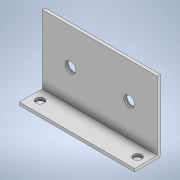
# Autodesk Inventor part: balun_support
Saved by Autodesk Inventor 2020.3 (Build 243373000, 373)
## iProperties
Created: 2021-03-09
Part Number: balun_support
Material: Generic
Document SubType Name: Modeling
Designer: Krishna Makhija
Density: 1 g/cm^3
Appearance: Default
Author: Krishna Makhija
Autodesk Inventor part; units mm, degrees
ref_plane "YZ Plane" through (0, 0, 0) normal (1, 0, 0) x (0, 1, 0)
ref_plane "XZ Plane" through (0, 0, 0) normal (0, 1, 0) x (-1, 0, 0)
ref_plane "XY Plane" through (0, 0, 0) normal (0, 0, 1) x (1, 0, 0)
sketch "Sketch1" plane through (0, 0, 0) normal (0, 0, 1) x (1, 0, 0)
  line L0 (29.994, -18.6437) -> (-29.994, -18.6437)
  line L1 (-29.994, 18.6437) -> (29.994, 18.6437)
  line L2 (29.994, -18.6437) -> (-29.994, 18.6437) construction
  line L3 (-29.994, -18.6437) -> (29.994, 18.6437) construction
  line L4 (29.994, -18.6437) -> (-29.994, -18.6437)
  line L5 (-29.994, -18.6437) -> (-29.994, -17.0588)
  line L6 (-29.994, -17.0588) -> (29.994, -17.0588)
  line L7 (29.994, -17.0588) -> (29.994, -18.6437)
  line L8 (-29.994, 18.6437) -> (-29.994, -17.0588)
  line L9 (29.994, 18.6437) -> (29.994, -17.0588)
  point P0 (0, 0)
  constraints: 20 end point, 3 parallel, 2 horizontal, 2 midpoint, 2 perpendicular, 1 vertical
extrude "Extrusion1" add sketch "Sketch1" against normal blind 1.5875 contours L6 L8 L1 L9
extrude "Extrusion2" add sketch "Sketch1" along normal blind 11.9062 and the other way blind 1.5875 contours L0 L5 L6 L7
sketch "Sketch2" plane through (-29.994, -17.0588, 0) normal (0, 1, 0) x (1, 0, 0)
  circle A0 centre (4.7625, -5.9531) radius 2.1855
  circle A1 centre (55.5625, -5.9531) radius 2.1855
  point P0 (29.994, 0)
  point P1 (0, 0)
  constraints: 2 centre point
sketch "Sketch3" plane through (0, 0, 0) normal (0, 0, 1) x (1, 0, 0)
  circle A0 centre (-15.2797, 0) radius 2.7871
  circle A1 centre (15.2797, 0) radius 2.7871
  constraints: 2 centre point
extrude "Extrusion3" cut sketch "Sketch3" against normal blind 25.4
extrude "Extrusion4" cut sketch "Sketch2" against normal blind 25.4
fillet "Fillet1" radius 1.5875 1 edges at (0, -18.6437, -1.5875)
body "Solid1"
